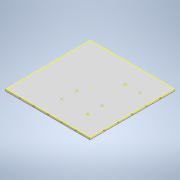
# Autodesk Inventor part: sheetmetalbottom2.0
Saved by Autodesk Inventor 2020.2 (Build 242310000, 310)
## iProperties
Created: 2020-02-06
Part Number: sheetmetalbottom2.0
Material: Generic
Document SubType Name: Modeling
Designer: ColinP
Density: 1 g/cm^3
Appearance: Default
Mass: 328.943 g
Surface Area: 1125.04 cm^2
Volume: 328.943 cm^3
Author: ColinP
Autodesk Inventor part; units mm, degrees
ref_plane "YZ Plane" through (0, 0, 0) normal (1, 0, 0) x (0, 1, 0)
ref_plane "XZ Plane" through (0, 0, 0) normal (0, 1, 0) x (-1, 0, 0)
ref_plane "XY Plane" through (0, 0, 0) normal (0, 0, 1) x (1, 0, 0)
sketch "Sketch1" plane through (0, 0, 0) normal (0, 1, 0) x (-1, 0, 0)
  line L0 (114.3, 114.3) -> (-114.3, 114.3)
  line L1 (-114.3, 114.3) -> (-114.3, -114.3)
  line L2 (-114.3, -114.3) -> (114.3, -114.3)
  line L3 (114.3, -114.3) -> (114.3, 114.3)
  point P0 (0, 0)
  dimension "d0" = 228.6
  dimension "d1" = 228.6
  constraints: 8 end point, 2 parallel, 1 horizontal, 1 perpendicular
  measures "d0" distance of L2.end L1.end
  measures "d1" distance of L1.end L0.end
extrude "Extrusion1" add sketch "Sketch1" along normal blind 6.35
sketch "Sketch2" plane through (114.3, 0, 114.3) normal (1, 0, 0) x (0, 0, -1)
  line L0 (0, 3.175) -> (38.1, 3.175)
  line L1 (38.1, 3.175) -> (76.2, 3.175)
  line L2 (76.2, 3.175) -> (114.3, 3.175)
  line L3 (114.3, 3.175) -> (152.4, 3.175)
  line L4 (152.4, 3.175) -> (190.5, 3.175)
  line L5 (190.5, 3.175) -> (228.6, 3.175)
  line L6 (228.6, 0) -> (228.6, 3.175)
  point P0 (114.3, 0)
  point P1 (0, 0)
  dimension "d4" = 38.1
  dimension "d5" = 38.1
  dimension "d6" = 38.1
  dimension "d7" = 38.1
  dimension "d8" = 38.1
  dimension "d85" = 3.175
  constraints: 14 end point, 4 point on line, 1 horizontal, 1 vertical
  measures "d4" distance of L0.start L0.end
  measures "d5" distance of L0.end L1.end
  measures "d6" distance of L1.end L2.end
  measures "d7" distance of L2.end L3.end
  measures "d8" distance of L3.end L4.end
  measures "d85" distance of L6.start L5.end
hole "Hole1" at (114.3, 3.175, 76.2) at (114.3, 3.175, 38.1) at (114.3, 3.175, 0) at (114.3, 3.175, -38.1) at (114.3, 3.175, -76.2) direction (-1, 0, 0) diameter 2.1565 depth 8.8646 thread size "4-40 UNC" class "2B" standard "ANSI Unified Screw Threads"
sketch "Sketch3" plane through (114.3, 0, -114.3) normal (0, 0, -1) x (-1, 0, 0)
  line L0 (0, 0) -> (0, 3.175)
  line L1 (0, 3.175) -> (38.1, 3.175)
  line L2 (38.1, 3.175) -> (76.2, 3.175)
  line L3 (76.2, 3.175) -> (114.3, 3.175)
  line L4 (114.3, 3.175) -> (152.4, 3.175)
  line L5 (152.4, 3.175) -> (190.5, 3.175)
  line L6 (190.5, 3.175) -> (228.6, 3.175)
  line L7 (228.6, 0) -> (228.6, 6.35) projected
  point P0 (114.3, 0)
  dimension "d16" = 38.1
  dimension "d17" = 38.1
  dimension "d18" = 38.1
  dimension "d19" = 38.1
  dimension "d20" = 38.1
  dimension "d83" = 3.175
  constraints: 14 end point, 4 point on line, 1 horizontal, 1 midpoint, 1 perpendicular
  measures "d16" distance of L0.end L1.end
  measures "d17" distance of L1.end L2.end
  measures "d18" distance of L2.end L3.end
  measures "d19" distance of L3.end L4.end
  measures "d20" distance of L4.end L5.end
  measures "d83" distance of L0.start L0.end
hole "Hole2" at (76.2, 3.175, -114.3) at (38.1, 3.175, -114.3) at (0, 3.175, -114.3) at (-38.1, 3.175, -114.3) at (-76.2, 3.175, -114.3) direction (0, 0, 1) diameter 2.1565 depth 8.8646 thread size "4-40 UNC" class "2B" standard "ANSI Unified Screw Threads"
sketch "Sketch4" plane through (-114.3, 0, -114.3) normal (-1, 0, 0) x (0, 0, 1)
  line L0 (0, 3.175) -> (38.1, 3.175)
  line L1 (38.1, 3.175) -> (76.2, 3.175)
  line L2 (76.2, 3.175) -> (114.3, 3.175)
  line L3 (114.3, 3.175) -> (152.4, 3.175)
  line L4 (152.4, 3.175) -> (190.5, 3.175)
  line L5 (0, 3.175) -> (0, 0)
  point P0 (114.3, 0)
  dimension "d28" = 38.1
  dimension "d29" = 38.1
  dimension "d30" = 38.1
  dimension "d31" = 38.1
  dimension "d32" = 38.1
  dimension "d86" = 3.175
  constraints: 12 end point, 4 point on line, 1 horizontal, 1 vertical
  measures "d28" distance of L0.start L0.end
  measures "d29" distance of L0.end L1.end
  measures "d30" distance of L1.end L2.end
  measures "d31" distance of L2.end L3.end
  measures "d32" distance of L3.end L4.end
  measures "d86" distance of L0.start L5.end
hole "Hole3" at (-114.3, 3.175, -76.2) at (-114.3, 3.175, -38.1) at (-114.3, 3.175, 0) at (-114.3, 3.175, 38.1) at (-114.3, 3.175, 76.2) direction (1, 0, 0) diameter 2.1565 depth 8.8646 thread size "4-40 UNC" class "2B" standard "ANSI Unified Screw Threads"
sketch "Sketch5" plane through (-114.3, 0, 114.3) normal (0, 0, 1) x (1, 0, 0)
  line L0 (0, 0) -> (0, 3.175)
  line L1 (0, 0) -> (0, 6.35) projected
  line L2 (0, 3.175) -> (38.1, 3.175)
  line L3 (0, 3.175) -> (38.1, 3.175) construction
  line L4 (38.1, 3.175) -> (76.2, 3.175)
  line L5 (76.2, 3.175) -> (114.3, 3.175)
  line L6 (114.3, 3.175) -> (152.4, 3.175)
  line L7 (152.4, 3.175) -> (190.5, 3.175)
  point P0 (114.3, 0)
  dimension "d40" = 3.175
  dimension "d41" = 38.1
  dimension "d42" = 0
  dimension "d43" = 38.1
  dimension "d44" = 38.1
  dimension "d45" = 38.1
  dimension "d46" = 38.1
  constraints: 14 end point, 4 point on line, 2 collinear, 2 horizontal
  measures "d40" distance of L0.start L0.end
  measures "d41" distance of L0.end L2.end
  measures "d42" distance between parallel lines of L2 L3
  measures "d43" distance of L2.end L4.end
  measures "d44" distance of L4.end L5.end
  measures "d45" distance of L5.end L6.end
  measures "d46" distance of L6.end L7.end
hole "Hole4" at (-76.2, 3.175, 114.3) at (-38.1, 3.175, 114.3) at (0, 3.175, 114.3) at (38.1, 3.175, 114.3) at (76.2, 3.175, 114.3) direction (0, 0, -1) diameter 2.1565 depth 8.8646 thread size "4-40 UNC" class "2B" standard "ANSI Unified Screw Threads"
sketch "Sketch6" plane through (0, 0, 0) normal (0, 1, 0) x (1, 0, 0)
  line L0 (-114.3, -114.3) -> (114.3, -114.3) projected
  line L1 (-114.3, -114.3) -> (-12.7, -114.3)
  line L2 (-12.7, -114.3) -> (-12.7, -63.5)
  line L3 (-12.7, -63.5) -> (-12.7, -23.622)
  line L4 (114.3, -114.3) -> (57.15, -114.3)
  line L5 (57.15, -114.3) -> (57.15, -63.5)
  line L6 (57.15, -63.5) -> (57.15, -23.622)
  line L7 (-114.3, 114.3) -> (-114.3, -114.3) projected
  line L8 (-114.3, 114.3) -> (-114.3, 57.15)
  line L9 (-114.3, 57.15) -> (38.1, 57.15)
  line L10 (38.1, 57.15) -> (77.978, 57.15)
  point P0 (0, 0)
  dimension "d54" = 101.6
  dimension "d55" = 50.8
  dimension "d56" = 39.878
  dimension "d57" = 57.15
  dimension "d58" = 57.15
  dimension "d59" = 152.4
  dimension "d60" = 39.878
  constraints: 18 end point, 6 point on line, 3 perpendicular
  measures "d54" distance of L0.start L1.end
  measures "d55" distance of L1.end L2.end
  measures "d56" distance of L2.end L3.end
  measures "d57" distance of L0.end L4.end
  measures "d58" distance of L7.start L8.end
  measures "d59" distance of L8.end L9.end
  measures "d60" distance of L9.end L10.end
hole "Hole5" at (77.978, 0, -57.15) at (38.1, 0, -57.15) at (-12.7, 0, 63.5) at (-12.7, 0, 23.622) at (57.15, 0, 23.622) at (57.15, 0, 63.5) direction (0, 1, 0) diameter 3.556 end through all countersink diameter 9.525 countersink angle 82
sketch "Sketch8" plane through (0, 6.35, 0) normal (0, 1, 0) x (1, 0, 0)
  circle A0 centre (57.15, -23.622) radius 1.778 projected
  circle A1 centre (-12.7, -63.5) radius 1.778 projected
  circle A2 centre (77.978, 57.15) radius 1.778 projected
  circle A3 centre (38.1, 57.15) radius 1.778 projected
  circle A4 centre (-12.7, -23.622) radius 1.778 projected
  circle A5 centre (57.15, -63.5) radius 1.778 projected
  line L0 (114.3, -114.3) -> (114.3, 114.3) projected
  line L1 (114.3, 114.3) -> (-114.3, 114.3) projected
  line L2 (-114.3, 114.3) -> (-114.3, -114.3) projected
  line L3 (-114.3, -114.3) -> (114.3, -114.3) projected
  point P0 (0, 0)
body "Solid1"
